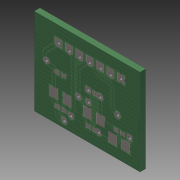
# Autodesk Inventor part: Sensor_module_envBoard
Saved by Autodesk Inventor 2013 (Build 170138000, 138)
## iProperties
Created: 2015-06-30
Part Number: Sensor_module_envBoard
Material: Ogólny
Document SubType Name: Modeling
Designer: terg
Density: 1 g/cm^3
Author: terg
Autodesk Inventor part; units mm, degrees
ref_plane "YZ Plane" through (0, 0, 0) normal (1, 0, 0) x (0, 1, 0)
ref_plane "XZ Plane" through (0, 0, 0) normal (0, 1, 0) x (-1, 0, 0)
ref_plane "XY Plane" through (0, 0, 0) normal (0, 0, 1) x (1, 0, 0)
sketch "Szkic1" plane through (0, 0, 0) normal (0, 1, 0) x (-1, 0, 0)
  line L0 (0, 0) -> (-15.25, 0)
  line L1 (-15.25, 0) -> (-15.25, 12.5)
  line L2 (-15.25, 12.5) -> (0, 12.5)
  line L3 (0, 12.5) -> (0, 0)
  dimension "d0" = 15.25
  dimension "d1" = 12.5
  constraints: 8 end point, 2 parallel, 1 horizontal, 1 perpendicular
  measures "d0" distance of L1.end L2.end
  measures "d1" distance of L0.end L1.end
extrude "Wyciągnięcie proste1" add sketch "Szkic1" along normal blind 0.8
sketch "Szkic2" plane through (0, 0.8, 0) normal (0, 1, 0) x (1, 0, 0)
  line L0 (0, 0) -> (15.211, 0.0473) construction
  line L1 (15.211, 0.0473) -> (15.25, -12.5) construction
  line L2 (15.25, -12.5) -> (0.039, -12.5473) construction
  line L3 (0.039, -12.5473) -> (0, 0) construction
  constraints: 2 other
decal "Pokrycie bitmapą1"
sketch "Szkic3" plane through (0, 0, 0) normal (0, -1, 0) x (1, 0, 0)
  line L0 (15.25, 0) -> (0.048, -0.0581) construction
  line L1 (0.048, -0.0581) -> (0, 12.5) construction
  line L2 (0, 12.5) -> (15.202, 12.5581) construction
  line L3 (15.202, 12.5581) -> (15.25, 0) construction
  constraints: 2 other
decal "Pokrycie bitmapą2"
sketch "Szkic4" plane through (0, 0, 0) normal (0, -1, 0) x (1, 0, 0)
  point P0 (3.4734, 10.2795)
  point P1 (5.0201, 10.0352)
  point P2 (6.5125, 10.0352)
  point P3 (7.9235, 10.0352)
  point P4 (9.531, 10.1492)
  point P5 (10.97, 10.0352)
  point P6 (12.4713, 10.319)
  point P7 (7.7305, 6.5261)
  point P8 (1.7193, 7.2236)
  point P9 (6.3228, 5.0296)
  point P10 (7.7939, 5.0296)
  point P11 (12.0043, 5.5369)
  point P12 (13.7291, 3.5078)
  point P13 (9.2545, 2.0022)
  point P14 (5.2493, 2.0657)
  point P15 (4.2829, 0.9676)
  point P16 (9.4856, 6.5261)
hole "Otwór1" at (3.4734, 0, 10.2795) at (5.0201, 0, 10.0352) at (6.5125, 0, 10.0352) at (7.9235, 0, 10.0352) at (9.531, 0, 10.1492) at (10.97, 0, 10.0352) at (12.4713, 0, 10.319) at (7.7305, 0, 6.5261) at (1.7193, 0, 7.2236) at (6.3228, 0, 5.0296) at (7.7939, 0, 5.0296) at (12.0043, 0, 5.5369) at (13.7291, 0, 3.5078) at (9.2545, 0, 2.0022) at (5.2493, 0, 2.0657) at (4.2829, 0, 0.9676) at (9.4856, 0, 6.5261) direction (0, 1, 0) diameter 0.4 depth 8
